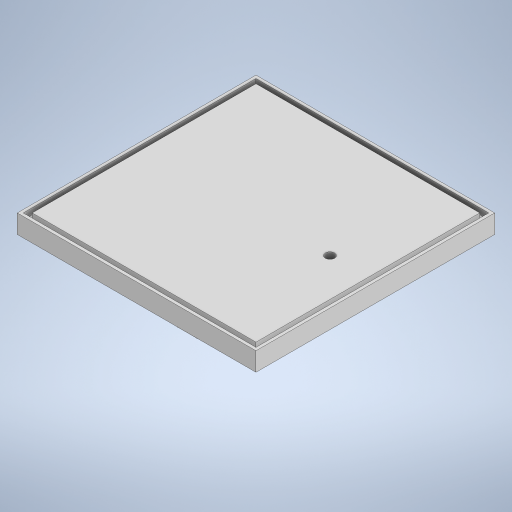
# Autodesk Inventor part: 사각형 OV-PAM 5패턴 상단
Saved by Autodesk Inventor 2024 (Build 280153000, 153)
## iProperties
Created: 2023-06-16
Part Number: 사각형 OV-PAM 5패턴 상단
Material: 일반
Document SubType Name: Modeling
Designer: jsw
Density: 1 g/cm^3
Appearance: 기본값
Author: jsw
Autodesk Inventor part; units mm, degrees
ref_plane "YZ Plane" through (0, 0, 0) normal (1, 0, 0) x (0, 1, 0)
ref_plane "XZ Plane" through (0, 0, 0) normal (0, 1, 0) x (-1, 0, 0)
ref_plane "XY Plane" through (0, 0, 0) normal (0, 0, 1) x (1, 0, 0)
sketch "스케치1" plane through (0, 0, 0) normal (0, 1, 0) x (-1, 0, 0)
  line L0 (0, 0) -> (64, 0)
  line L1 (64, 0) -> (64, -64)
  line L2 (64, -64) -> (0, -64)
  line L3 (0, -64) -> (0, 0)
  dimension "d0" = 64
  dimension "d1" = 64
  constraints: 8 end point, 2 parallel, 1 horizontal, 1 perpendicular
  measures "d0" distance of L2.end L0.start
  measures "d1" distance of L0.start L0.end
extrude "돌출1" add sketch "스케치1" along normal blind 5
sketch "스케치2" plane through (0, 5, 0) normal (0, 1, 0) x (1, 0, 0)
  line L0 (-2, 2) -> (-62, 2)
  line L1 (-62, 2) -> (-62, 62)
  line L2 (-62, 62) -> (-2, 62)
  line L3 (-2, 62) -> (-2, 2)
  line L4 (-64, 0) -> (0, 0) projected
  line L5 (0, 0) -> (0, 64) projected
  line L6 (-63.2, 0.8) -> (-0.8, 0.8)
  line L7 (-0.8, 0.8) -> (-0.8, 63.2)
  line L8 (-0.8, 63.2) -> (-63.2, 63.2)
  line L9 (-63.2, 63.2) -> (-63.2, 0.8)
  dimension "d4" = 60
  dimension "d5" = 60
  dimension "d6" = 2
  dimension "d7" = 2
  dimension "d8" = 1.2
  dimension "d9" = 1.2
  dimension "d37" = 1.2
  dimension "d38" = 1.2
  constraints: 16 end point, 4 parallel, 2 horizontal, 2 perpendicular
  measures "d4" distance of L0.end L1.end
  measures "d5" distance of L1.end L2.end
  measures "d6" distance between parallel lines of L4 L0
  measures "d7" distance between parallel lines of L5 L3
  measures "d8" distance between parallel lines of L9 L1
  measures "d9" distance between parallel lines of L8 L2
  measures "d37" distance between parallel lines of L6 L0
  measures "d38" distance between parallel lines of L3 L7
extrude "돌출2" cut sketch "스케치2" against normal blind 1.6
sketch "스케치3" plane through (0, 0, 0) normal (0, -1, 0) x (1, 0, 0)
  line L0 (-29.5, -12) -> (-34.5, -12)
  line L1 (-34.5, -12) -> (-34.5, -22)
  line L2 (-34.5, -22) -> (-29.5, -22)
  line L3 (-29.5, -22) -> (-29.5, -12)
  line L4 (-64, 0) -> (0, 0) projected
  line L5 (-29.5, -42) -> (-34.5, -42)
  line L6 (-34.5, -42) -> (-34.5, -52)
  line L7 (-34.5, -52) -> (-29.5, -52)
  line L8 (-29.5, -52) -> (-29.5, -42)
  line L9 (0, -64) -> (-64, -64) projected
  line L10 (-2, -62) -> (-62, -62) projected
  point P0 (-32, -12)
  point P1 (-32, 0)
  point P2 (-32, -42)
  point P3 (-32, -52)
  dimension "d12" = 10
  dimension "d13" = 5
  dimension "d16" = 30
  dimension "d22" = 10
  constraints: 16 end point, 3 midpoint, 2 parallel, 1 collinear, 1 horizontal, 1 perpendicular, 1 vertical, 1 vertical alignment, 8 other
  measures "d12" distance of L2.end L0.start
  measures "d13" distance of L0.start L0.end
  measures "d16" distance of L0.start L5.start
  measures "d22" distance from line of point (-32, -52) L10
extrude "돌출3" add sketch "스케치3" along normal blind 10
sketch "스케치4" plane through (-34.5, 0, -22) normal (-1, 0, 0) x (0, 0, 1)
  line L0 (10, -10) -> (0, -10) projected
  circle A0 centre (5, -10) radius 5
  line L1 (-30, -10) -> (-20, -10) projected
  circle A1 centre (-25, -10) radius 5
  point P0 (22, 0)
  dimension "d25" = 10
  dimension "d26" = 10
  constraints: 2 centre point, 2 midpoint
  measures "d25" diameter of A0
  measures "d26" diameter of A1
extrude "돌출4" add sketch "스케치4" against normal blind 5
sketch "스케치5" plane through (-34.5, 0, -22) normal (-1, 0, 0) x (0, 0, 1)
  arc A0 (0, -10) -> (10, -10) centre (5, -10) ccw projected
  circle A1 centre (5, -10) radius 1.25
  arc A2 (-30, -10) -> (-20, -10) centre (-25, -10) ccw projected
  circle A3 centre (-25, -10) radius 1.25
  point P0 (22, 0)
  dimension "d29" = 2.5
  dimension "d30" = 2.5
  constraints: 2 centre point, 2 coincident
  measures "d29" diameter of A1
  measures "d30" diameter of A3
extrude "돌출5" cut sketch "스케치5" against normal blind 5
sketch "스케치6" plane through (0, 0, 0) normal (0, -1, 0) x (1, 0, 0)
  circle A0 centre (-12.179, -32) radius 1.25
  line L0 (0, 0) -> (0, -64) projected
  line L1 (-29.5, -12) -> (-29.5, -22) projected
  point P0 (0, -32)
  dimension "d33" = 2.5
  dimension "d34" = 17.321
  constraints: 1 centre point, 1 horizontal alignment, 1 midpoint
  measures "d33" diameter of A0
  measures "d34" distance from line of L1 A0.centre
extrude "돌출6" cut sketch "스케치6" against normal blind 5
